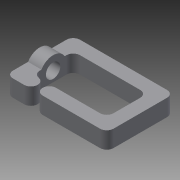
# Autodesk Inventor part: CounterWeightHook
Saved by Autodesk Inventor 2014 SP1 (Build 180222100, 222)
## iProperties
Created: 2017-02-25
Part Number: CounterWeightHook
Material: Generic
Document SubType Name: Modeling
Designer: danielsikar
Density: 1 g/cm^3
Appearance: Default
Author: danielsikar
Autodesk Inventor part; units mm, degrees
ref_plane "YZ Plane" through (0, 0, 0) normal (1, 0, 0) x (0, 1, 0)
ref_plane "XZ Plane" through (0, 0, 0) normal (0, 1, 0) x (-1, 0, 0)
ref_plane "XY Plane" through (0, 0, 0) normal (0, 0, 1) x (1, 0, 0)
sketch "Sketch1" plane through (0, 0, 0) normal (0, 0, 1) x (1, 0, 0)
  line L0 (0, 0) -> (30, 0)
  line L1 (30, 0) -> (30, 20)
  line L2 (30, 20) -> (0, 20)
  line L3 (0, 20) -> (0, 0)
  dimension "d0" = 30
  dimension "d1" = 20
  constraints: 8 end point, 2 parallel, 1 horizontal, 1 perpendicular
  measures "d0" distance of L2.end L1.end
  measures "d1" distance of L1.end L0.end
extrude "Extrusion1" add sketch "Sketch1" along normal blind 5
sketch "Sketch2" plane through (0, 0, 5) normal (0, 0, 1) x (1, 0, 0)
  line L0 (30, 20) -> (0, 20) projected
  line L1 (0, 20) -> (0, 0) projected
  line L2 (4, 16) -> (26, 16)
  line L3 (26, 16) -> (26, 4)
  line L4 (26, 4) -> (4, 4)
  line L5 (4, 4) -> (4, 16)
  point P0 (15, 16)
  point P1 (15, 20)
  point P2 (4, 10)
  point P3 (0, 10)
  dimension "d4" = 22
  dimension "d5" = 12
  constraints: 8 end point, 4 midpoint, 2 parallel, 1 horizontal, 1 horizontal alignment, 1 perpendicular, 1 vertical alignment
  measures "d4" distance of L3.end L4.end
  measures "d5" distance of L2.end L3.end
extrude "Extrusion2" cut sketch "Sketch2" against normal blind 5
sketch "Sketch3" plane through (4, 4, 5) normal (1, 0, 0) x (0, 0, -1)
  line L0 (0, 0) -> (0, 12) projected
  line L1 (5, 12) -> (5, 0) projected
  arc A0 (0, 5.211) -> (0, 6.789) centre (2, 6) ccw
  circle A1 centre (2, 6) radius 4
  line L2 (5, 2.5413) -> (5, 9.5535)
  line L3 (0, 10.4236) -> (0, 1.364)
  point P0 (5, -4)
  dimension "d8" = 4.3
  dimension "d9" = 8
  constraints: 6 point on line, 4 end point, 2 centre point, 2 point on circle, 1 coincident
  measures "d8" diameter of A0
  measures "d9" diameter of A1
extrude "Extrusion3" add sketch "Sketch3" against normal blind 4 contours L0 A1 | A0 L0 A1 L1 | L1 A1
sketch "Sketch4" plane through (0, 20, 0) normal (-1, 0, 0) x (0, 0, 1)
  arc A0 (5, -13.4641) -> (5, -6.5359) centre (3, -10) ccw projected
  circle A1 centre (3, -10) radius 2.15
  dimension "d12" = 4.3
  constraints: 1 centre point, 1 coincident
  measures "d12" diameter of A1
extrude "Extrusion4" cut sketch "Sketch4" against normal blind 4
sketch "Sketch5" plane through (0, 20, 0) normal (-1, 0, 0) x (0, 0, 1)
  line L0 (5, 0) -> (5, -6.5359) projected
  line L1 (0, 0) -> (5, 0) projected
  line L2 (0, 0) -> (0, -7.3542) projected
  arc A0 (0, -7.3542) -> (0, -12.6458) centre (3, -10) ccw projected
  line L3 (0, -12.6458) -> (0, -20) projected
  line L4 (0, -20) -> (5, -20) projected
  line L5 (5, -13.4641) -> (5, -20) projected
  arc A1 (5, -13.4641) -> (5, -6.5359) centre (3, -10) ccw projected
  line L6 (0, -5.3679) -> (0, -13.4641)
  arc A2 (0, -7.3542) -> (0, -12.6458) centre (3, -10) ccw
  constraints: 2 end point, 2 point on circle, 2 point on line, 1 centre point, 1 concentric
extrude "Extrusion5" cut sketch "Sketch5" against normal blind 4 contours L6 A0
sketch "Sketch6" plane through (0, 0, 0) normal (0, 0, -1) x (-1, 0, 0)
  line L0 (-4, 4) -> (-26, 4) projected
  line L1 (0, 0) -> (-30, 0) projected
  line L2 (-7.3617, 4) -> (-8.8617, 4)
  line L3 (-8.8617, 4) -> (-8.8617, 0)
  line L4 (-8.8617, 0) -> (-7.3617, 0)
  line L5 (-7.3617, 0) -> (-7.3617, 4)
  dimension "d17" = 1.5
  constraints: 8 end point, 2 parallel, 2 point on line, 1 horizontal, 1 perpendicular
  measures "d17" distance of L4.end L3.end
extrude "Extrusion6" cut sketch "Sketch6" against normal blind 5
fillet "Fillet1" radius 2 12 edges at (0, 0, 2.5) (0, 20, 2.5) (30, 0, 2.5) (30, 20, 2.5) (26, 16, 2.5) (26, 4, 2.5) (4, 4, 2.5) (4, 16, 2.5) (8.8617, 0, 2.5) (8.8617, 4, 2.5) (7.3617, 0, 2.5) (7.3617, 4, 2.5)
body "Solid1"
